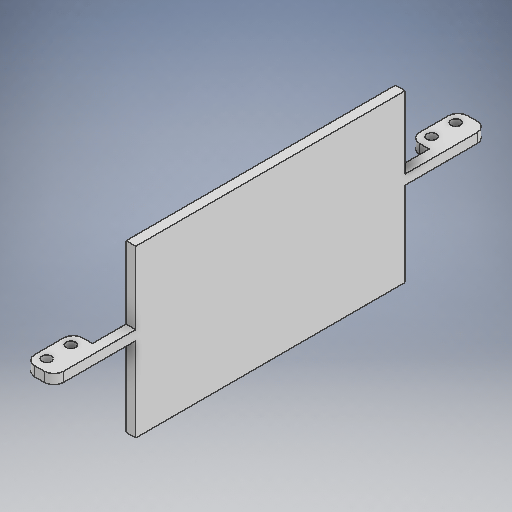
# Autodesk Inventor part: rigid_support2
Saved by Autodesk Inventor 2026.1 (Build 301233000, 233)
## iProperties
Created: 2025-10-27
Part Number: rigid_support2
Material: Generic
Document SubType Name: Modeling
Designer: emanuel
Density: 1 g/cm^3
Appearance: Default
Author: emanuel
Autodesk Inventor part; units mm, degrees
ref_plane "YZ Plane" through (0, 0, 0) normal (1, 0, 0) x (0, 1, 0)
ref_plane "XZ Plane" through (0, 0, 0) normal (0, 1, 0) x (-1, 0, 0)
ref_plane "XY Plane" through (0, 0, 0) normal (0, 0, 1) x (1, 0, 0)
sketch "Sketch1" plane through (0, 0, 0) normal (0, 1, 0) x (-1, 0, 0)
  line L0 (0, 0) -> (8, 0)
  line L1 (8, 0) -> (8, 20)
  line L2 (8, 20) -> (0, 20)
  line L3 (0, 20) -> (0, 0)
  line L4 (8, 20) -> (4, 20)
  line L5 (4, 20) -> (4, 15)
  line L6 (4, 15) -> (8, 15)
  line L7 (8, 15) -> (8, 20)
  line L8 (4, 15) -> (4, 5)
  circle A0 centre (4, 15) radius 2
  circle A1 centre (4, 5) radius 2
  line L9 (0, 20) -> (-4, 20)
  line L10 (-4, 20) -> (-4, -70)
  line L11 (-4, -70) -> (0, -70)
  line L12 (0, -70) -> (0, 20)
  line L13 (0, -140) -> (8, -140)
  line L14 (8, -140) -> (8, -160)
  line L15 (8, -160) -> (0, -160)
  line L16 (0, -160) -> (0, -140)
  line L17 (8, -160) -> (4, -160)
  line L18 (4, -160) -> (4, -155)
  line L19 (4, -155) -> (8, -155)
  line L20 (8, -155) -> (8, -160)
  line L21 (4, -155) -> (4, -145)
  circle A2 centre (4, -155) radius 2
  circle A3 centre (4, -145) radius 2
  line L22 (0, -160) -> (-4, -160)
  line L23 (-4, -160) -> (-4, -70)
  line L24 (0, -70) -> (0, -160)
  dimension "d0" = 8
  dimension "d1" = 20
  dimension "d2" = 4
  dimension "d3" = 5
  dimension "d4" = 10
  dimension "d5" = 4
  dimension "d6" = 4
  constraints: 50 end point, 11 symmetric about line, 6 parallel, 4 centre point, 4 coincident, 3 horizontal, 3 perpendicular, 1 vertical, 2 other
  measures "d0" distance of L2.end L1.end
  measures "d1" distance of L0.end L1.end
  measures "d2" distance of L6.end L5.end
  measures "d3" distance of L5.end L4.end
  measures "d4" distance of L5.end L8.end
  measures "d5" diameter of A0
  measures "d6" diameter of A1
extrude "Extrusion1" add sketch "Sketch1" along normal blind 4 contours L3 L2 L5 A0 L6 L1 L0 | L12 L11 L10 L9 L3 | L24 L16 L22 L23 L11 | L6 A0 L5 L2 L1 | L13 L14 L19 A2 L18 L15 L16 | L14 L15 L18 A2 L19
fillet "Fillet1" radius 4 6 edges at (-8, 2, -140) (-8, 2, -160) (4, 2, -160) (4, 2, 20) (-8, 2, 20) (-8, 2, 0)
sketch "Sketch2" plane through (4, 0, 16) normal (1, 0, 0) x (0, 0, -1)
  line L0 (-4, 4) -> (0, 4) projected
  line L1 (0, 4) -> (30, 4)
  line L2 (156, 4) -> (16, 4) projected
  line L3 (172, 4) -> (172, 0) projected
  line L4 (172, 4) -> (142, 4)
  line L5 (30, 4) -> (142, 4)
  line L6 (142, 4) -> (142, 34)
  line L7 (142, 34) -> (30, 34)
  line L8 (30, 34) -> (30, 4)
  line L9 (156, 0) -> (16, 0) projected
  line L10 (30, 0) -> (142, 0)
  line L11 (142, 0) -> (142, -35)
  line L12 (142, -35) -> (30, -35)
  line L13 (30, -35) -> (30, 0)
  dimension "d12" = 30
  dimension "d13" = 30
  dimension "d14" = 30
  dimension "d15" = 35
  constraints: 20 end point, 4 parallel, 3 point on line, 2 horizontal, 2 perpendicular
  measures "d12" distance of L0.end L1.end
  measures "d13" distance of L3.start L4.end
  measures "d14" distance of L6.end L5.end
  measures "d15" distance of L10.end L11.end
extrude "Extrusion2" add sketch "Sketch2" against normal up to surface (4 mm away)
body "Solid1"
